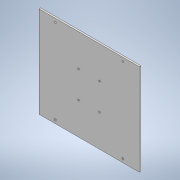
# Autodesk Inventor part: side plate
Saved by Autodesk Inventor 2021 (Build 250183000, 183)
## iProperties
Created: 2021-06-03
Part Number: side plate
Material: Generic
Document SubType Name: Modeling
Designer: capta
Density: 1 g/cm^3
Appearance: Default
Author: capta
Autodesk Inventor part; units mm, degrees
ref_plane "YZ Plane" through (0, 0, 0) normal (1, 0, 0) x (0, 1, 0)
ref_plane "XZ Plane" through (0, 0, 0) normal (0, 1, 0) x (-1, 0, 0)
ref_plane "XY Plane" through (0, 0, 0) normal (0, 0, 1) x (1, 0, 0)
sketch "Sketch1" plane through (0, 0, 0) normal (0, 0, 1) x (1, 0, 0)
  line L0 (-88.9, -80.9625) -> (88.9, -80.9625)
  line L1 (88.9, -80.9625) -> (88.9, 80.9625)
  line L2 (88.9, 80.9625) -> (-88.9, 80.9625)
  line L3 (-88.9, 80.9625) -> (-88.9, -80.9625)
  line L4 (-88.9, -80.9625) -> (88.9, 80.9625) construction
  line L5 (88.9, -80.9625) -> (-88.9, 80.9625) construction
  point P0 (0, 0)
  dimension "d0" = 177.8
  dimension "d1" = 161.925
  constraints: 12 end point, 2 midpoint, 2 parallel, 1 horizontal, 1 perpendicular
  measures "d0" distance of L1.end L2.end
  measures "d1" distance of L0.end L1.end
extrude "Extrusion1" add sketch "Sketch1" along normal blind 3.048
sketch "Sketch2" plane through (0, 0, 3.048) normal (0, 0, 1) x (1, 0, 0)
  line L0 (-59.817, -74.676) -> (59.817, -74.676)
  line L1 (59.817, -74.676) -> (59.817, 74.676)
  line L2 (59.817, 74.676) -> (-59.817, 74.676)
  line L3 (-59.817, 74.676) -> (-59.817, -74.676)
  line L4 (-59.817, -74.676) -> (59.817, 74.676) construction
  line L5 (59.817, -74.676) -> (-59.817, 74.676) construction
  point P0 (0, 0)
  dimension "d4" = 119.634
  dimension "d5" = 149.352
  constraints: 12 end point, 4 coincident, 2 midpoint, 2 parallel, 1 horizontal, 1 perpendicular
  measures "d4" distance of L1.end L2.end
  measures "d5" distance of L0.end L1.end
hole "Hole1" at (-59.817, 74.676, 3.048) at (-59.817, -74.676, 3.048) at (59.817, -74.676, 3.048) at (59.817, 74.676, 3.048) direction (0, 0, -1) diameter 3.048 end through all
sketch "Sketch3" plane through (0, 0, 3.048) normal (0, 0, 1) x (1, 0, 0)
  line L0 (-18.542, -23.876) -> (18.542, -23.876)
  line L1 (18.542, -23.876) -> (18.542, 23.876)
  line L2 (18.542, 23.876) -> (-18.542, 23.876)
  line L3 (-18.542, 23.876) -> (-18.542, -23.876)
  line L4 (-18.542, -23.876) -> (18.542, 23.876) construction
  line L5 (18.542, -23.876) -> (-18.542, 23.876) construction
  point P0 (0, 0)
  dimension "d13" = 37.084
  dimension "d14" = 47.752
  constraints: 12 end point, 4 coincident, 2 midpoint, 2 parallel, 1 horizontal, 1 perpendicular
  measures "d13" distance of L1.end L2.end
  measures "d14" distance of L0.end L1.end
hole "Hole2" at (-18.542, 23.876, 3.048) at (18.542, 23.876, 3.048) at (18.542, -23.876, 3.048) at (-18.542, -23.876, 3.048) direction (0, 0, -1) diameter 2.7432 end through all
body "Solid1"
